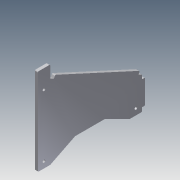
# Autodesk Inventor part: LeftSidePanel
Saved by Autodesk Inventor 2014 (Build 180170000, 170)
## iProperties
Created: 2015-01-19
Part Number: LeftSidePanel
Material: Generic
Document SubType Name: Modeling
Designer: Peele
Density: 1 g/cm^3
Appearance: White
Author: Peele
Autodesk Inventor part; units mm, degrees
ref_plane "YZ Plane" through (0, 0, 0) normal (1, 0, 0) x (0, 1, 0)
ref_plane "XZ Plane" through (0, 0, 0) normal (0, 1, 0) x (-1, 0, 0)
ref_plane "XY Plane" through (0, 0, 0) normal (0, 0, 1) x (1, 0, 0)
sketch "Sketch1" plane through (0, 0, 0) normal (1, 0, 0) x (0, 1, 0)
  line L0 (0, 0) -> (0, 175)
  line L1 (0, 175) -> (25, 175)
  line L2 (25, 175) -> (25, 150)
  line L3 (210, 65) -> (210, 0)
  line L4 (210, 0) -> (0, 0)
  line L5 (25, 150) -> (210, 65)
  line L6 (210, 65) -> (210, 150) construction
  line L7 (210, 150) -> (25, 150) construction
  dimension "d0" = 175
  dimension "d1" = 25
  dimension "d3" = 65
  dimension "d4" = 210
  dimension "d27" = 185
  dimension "d28" = 85
  constraints: 16 end point, 3 parallel, 3 perpendicular, 1 vertical
  measures "d0" distance of L0.start L0.end
  measures "d1" distance of L0.end L1.end
  measures "d3" distance of L3.start L3.end
  measures "d4" distance of L3.end L0.start
  measures "d27" distance of L2.end L6.end
  measures "d28" distance of L3.start L6.end
extrude "Extrusion1" add sketch "Sketch1" along normal blind 6
sketch "Sketch2" plane through (6, 0, 0) normal (1, 0, 0) x (0, 0, -1)
  line L0 (0, 0) -> (0, 210) projected
  line L1 (0, 210) -> (-65, 210) projected
  line L2 (-175, 0) -> (0, 0) projected
  line L3 (0, 185) -> (-25, 135)
  line L4 (-25, 135) -> (-25, 75)
  line L5 (-25, 75) -> (0, 25)
  line L6 (0, 185) -> (0, 25)
  dimension "d8" = 25
  dimension "d9" = 25
  dimension "d10" = 50
  dimension "d11" = 25
  constraints: 8 end point, 2 point on line, 1 equal length, 1 parallel, 1 perpendicular
  measures "d8" distance between parallel lines of L6 L4
  measures "d9" distance from line of L5.end L2
  measures "d10" vertical distance of L4.end L5.end
  measures "d11" distance from line of L3.start L1
extrude "Extrusion2" cut sketch "Sketch2" against normal through all
sketch "Sketch3" plane through (6, 0, 0) normal (1, 0, 0) x (0, 0, -1)
  line L0 (0, 185) -> (0, 210) projected
  line L1 (0, 210) -> (-65, 210) projected
  line L2 (-56.9, 210) -> (-8.1, 210)
  line L3 (-8.1, 210) -> (-8.1, 216)
  line L4 (-8.1, 216) -> (-56.9, 216)
  line L5 (-56.9, 216) -> (-56.9, 210)
  dimension "d14" = 8.1
  dimension "d15" = 8.1
  dimension "d16" = 6
  constraints: 8 end point, 2 parallel, 1 horizontal, 1 perpendicular, 1 point on line
  measures "d14" distance between parallel lines of L3 L0
  measures "d15" distance from line of L1.end L5
  measures "d16" distance of L2.end L3.end
extrude "Extrusion3" add sketch "Sketch3" against normal blind 6
sketch "Sketch4" plane through (6, 0, 0) normal (1, 0, 0) x (0, 0, -1)
  line L0 (0, 210) -> (-8.1, 210) projected
  line L1 (-175, 25) -> (-175, 0) projected
  line L2 (-175, 0) -> (0, 0) projected
  line L3 (0, 0) -> (0, 25) projected
  circle A0 centre (-12.5, 197.5) radius 2.7
  circle A1 centre (-12.5, 12.5) radius 2.7
  circle A2 centre (-137.5, 12.5) radius 2.7
  dimension "d19" = 12.5
  dimension "d20" = 37.5
  dimension "d21" = 12.5
  dimension "d22" = 12.5
  dimension "d23" = 5.4
  constraints: 3 centre point, 2 equal radius, 1 horizontal alignment, 1 vertical alignment
  measures "d19" distance from line of A2.centre L2
  measures "d20" distance from line of A2.centre L1
  measures "d21" distance from line of A1.centre L3
  measures "d22" distance from line of A0.centre L0
  measures "d23" diameter of A0
extrude "Extrusion4" cut sketch "Sketch4" against normal through all
sketch "Sketch6" plane through (6, 0, 0) normal (1, 0, 0) x (0, 0, -1)
  line L0 (-65, 210) -> (-150, 25) projected
  line L1 (-146.6182, 32.3603) -> (-152.0703, 34.8653)
  line L2 (-152.0703, 34.8653) -> (-73.8338, 205.1447)
  line L3 (-73.8338, 205.1447) -> (-68.3818, 202.6397)
  line L4 (-146.6182, 32.3603) -> (-68.3818, 202.6397)
  dimension "d33" = 8.1
  dimension "d36" = 8.1
  dimension "d38" = 6
  constraints: 8 end point, 4 perpendicular, 2 point on line
  measures "d33" distance from line of L0.start L3
  measures "d36" distance from line of L0.end L1
  measures "d38" distance between parallel lines of L2 L0
extrude "Extrusion5" add sketch "Sketch6" against normal blind 6
fillet "Fillet1" radius 2 14 edges at (3, 25, 175) (3, 0, 175) (3, 25, 150) (3, 210, 65) (3, 216, 56.9) (3, 216, 8.1) (3, 210, 0) (3, 185, 0) (3, 135, 25) (3, 75, 25) (3, 25, 0) (3, 0, 0) (3, 34.8653, 152.0703) (3, 205.1447, 73.8338)
equation "\"d11\" = d9"
equation "\"d15\" = d14"
body "Solid1"
